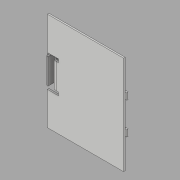
# Autodesk Inventor part: BAcA_3
Saved by Autodesk Inventor 2019.3 (Build 233278000, 278)
## iProperties
Created: 2019-02-21
Part Number: BAcA_3
Material: Generic
Document SubType Name: Modeling
Designer: Varga Daniel
Density: 1 g/cm^3
Appearance: Default
Author: Varga Daniel
Autodesk Inventor part; units mm, degrees
ref_plane "YZ Plane" through (0, 0, 0) normal (1, 0, 0) x (0, 1, 0)
ref_plane "XZ Plane" through (0, 0, 0) normal (0, 1, 0) x (-1, 0, 0)
ref_plane "XY Plane" through (0, 0, 0) normal (0, 0, 1) x (1, 0, 0)
ref_plane "Work Plane1" through (0, 0, 0) normal (0, 0, 1) x (1, 0, 0)
sketch "Sketch1" plane through (0, 0, 0) normal (0, 0, 1) x (1, 0, 0)
  line L0 (-60, -72.111) -> (-60, -152.111) construction
  line L1 (0, -152.111) -> (-60, -152.111) construction
  line L2 (0, -72.111) -> (0, -152.111) construction
  line L3 (0, -72.111) -> (-60, -72.111) construction
  line L4 (-9.2, -81.311) -> (-57, -81.311) construction
  line L5 (-9.2, -142.911) -> (-9.2, -81.311) construction
  line L6 (-57, -142.911) -> (-9.2, -142.911) construction
  line L7 (-57, -81.311) -> (-57, -142.911) construction
  line L8 (-57, -81.311) -> (-9.2, -81.311)
  line L9 (-9.2, -81.311) -> (-9.2, -142.911)
  line L10 (-9.2, -142.911) -> (-57, -142.911)
  line L11 (-57, -142.911) -> (-57, -81.311)
  line L12 (-57, -112.111) -> (-9.2, -112.111) construction
  line L13 (-57, -102.111) -> (-50, -102.111)
  line L14 (-50, -102.111) -> (-50, -122.111)
  line L15 (-50, -122.111) -> (-57, -122.111)
  line L16 (-57, -122.111) -> (-57, -102.111)
  point P0 (0, 0)
  dimension "d0" = 20
  dimension "d1" = 7
  constraints: 18 end point, 5 parallel, 2 horizontal, 2 midpoint, 2 perpendicular, 1 point on line, 2 other
  measures "d0" distance between parallel lines of L15 L13
  measures "d1" distance between parallel lines of L16 L14
extrude "Extrusion1" add sketch "Sketch1" against normal blind 1 contours L8 L9 L10 L11 L15 L14 L13
ref_plane "Work Plane2" through (-57, -112.111, 0) normal (0, 1, 0) x (1, 0, 0)
sketch "Sketch2" plane through (-57, -112.111, 0) normal (0, 1, 0) x (1, 0, 0)
  line L0 (7, 0) -> (0, 0) construction
  line L1 (7, 0) -> (7, 1) construction
  line L2 (0, 1) -> (7, 1) construction
  line L3 (0, 0) -> (0, 1) construction
  line L4 (-0.5921, 0.3244) -> (-0.4121, 1.1039)
  line L5 (-0.4121, 1.1039) -> (-1.3865, 1.3289)
  line L6 (-1.3865, 1.3289) -> (-0.4744, 5.2798)
  arc A0 (1.3347, 5.6055) -> (-0.4744, 5.2798) centre (0.5, 5.0549) ccw
  line L7 (1.3347, 5.6055) -> (3.7801, 1.8987)
  arc A1 (3.7801, 1.8987) -> (5.4496, 1) centre (5.4496, 3) ccw
  line L8 (5.4496, 1) -> (7, 1)
  line L9 (7, 1) -> (7, 0)
  line L10 (7, 0) -> (5.4496, 0)
  arc A2 (2.9454, 1.348) -> (5.4496, 0) centre (5.4496, 3) ccw
  line L11 (2.9454, 1.348) -> (0.5436, 4.9888)
  arc A3 (0.5436, 4.9888) -> (0.4529, 4.9616) centre (0.5023, 4.9616) ccw
  line L12 (47.8, 0) -> (0, 0) projected
  line L13 (47.8, 1) -> (0, 1) projected
  line L14 (5.4496, 0) -> (5.4496, 1) construction
  line L15 (0.4529, 0.1293) -> (0.4529, 4.9616)
  line L16 (-0.4422, 0.0846) -> (0.2079, -0.0655)
  arc A4 (0.2079, -0.0655) -> (0.4529, 0.1293) centre (0.2529, 0.1293) ccw
  arc A5 (-0.5921, 0.3244) -> (-0.4422, 0.0846) centre (-0.3972, 0.2794) ccw
  point P0 (57, 0)
  point P1 (0.4529, -0.1221)
  point P2 (-0.6371, 0.1296)
  dimension "d8" = 1
  dimension "d9" = 1
  dimension "d11" = 1
  dimension "d12" = 0.0494
  dimension "d22" = 1
  dimension "d23" = 2
  dimension "d31" = 13
  dimension "d32" = 1
  dimension "d33" = 4.0549
  dimension "d34" = 2.1187
  dimension "d35" = 4.4408
  dimension "d36" = 0.2
  constraints: 20 end point, 12 point on circle, 12 tangent, 6 centre point, 4 point on line, 3 parallel, 2 collinear, 1 equal radius, 1 horizontal, 1 perpendicular, 8 other
  measures "d8" distance between parallel lines of L11 L7
  measures "d9" distance between parallel lines of L8 L10
  measures "d11" radius of A0
  measures "d12" radius of A3
  measures "d22" distance from line of L4 L6.start
  measures "d23" radius of A1
  measures "d31" angle of L6 L15
  measures "d34" distance from line of point (0.453, -0.122) L6
  measures "d35" distance of L7.start L7.end
  measures "d36" radius of A4
extrude "Extrusion2" add sketch "Sketch2" along normal mid plane 16 contours L4 L5 L6 A0 L7 A1 L13 A2 L11 A3 L15 A4 L16 A5 | A2 L13 L8 L9 L10
ref_plane "Work Plane3" through (-57, -102.111, 0) normal (0, 1, 0) x (1, 0, 0)
sketch "Sketch4" plane through (-57, -102.111, 0) normal (0, 1, 0) x (1, 0, 0)
  line L0 (57, 0) -> (-3, 0) construction
  line L1 (0, 0) -> (47.8, 0) construction
  line L2 (47.8, 0) -> (47.8, 1) construction
  line L3 (0, 1) -> (47.8, 1) construction
  line L4 (0, 0) -> (0, 1) construction
  line L5 (0, 1) -> (47.8, 1) projected
  line L6 (46.8, 1) -> (47.8, 1)
  line L7 (47.8, 1) -> (48.8, 1)
  line L8 (48.8, 1) -> (48.8, 1.6)
  line L9 (48.4, 2) -> (47.2, 2)
  line L10 (46.8, 1.6) -> (46.8, 1)
  arc A0 (48.8, 1.6) -> (48.4, 2) centre (48.4, 1.6) ccw
  arc A1 (47.2, 2) -> (46.8, 1.6) centre (47.2, 1.6) ccw
  point P0 (48.8, 2)
  dimension "d25" = 1
  dimension "d26" = 1
  dimension "d27" = 1
  dimension "d28" = 0.4
  constraints: 10 end point, 4 point on circle, 4 point on line, 4 tangent, 3 perpendicular, 2 centre point, 1 collinear, 1 equal radius
  measures "d25" distance of L7.end point (48.8, 2)
  measures "d26" distance between parallel lines of L2 L8
  measures "d27" distance between parallel lines of L2 L10
  measures "d28" radius of A0
extrude "Extrusion3" add sketch "Sketch4" along normal mid plane 4
mirror "Mirror1" about plane through (-57, -112.111, 0) normal (0, 1, 0) of "Extrusion3"
equation "\"d8\" = d9"
body "Solid1"
